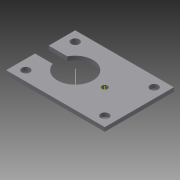
# Autodesk Inventor part: GehäuseFront
Saved by Autodesk Inventor 2014 (Build 180170000, 170)
## iProperties
Created: 2013-05-31
Part Number: GehäuseFront
Material: Generisch
Document SubType Name: Modeling
Designer: hanse
Density: 1 g/cm^3
Appearance: Vorgabe
Author: hanse
Autodesk Inventor part; units mm, degrees
ref_plane "YZ Plane" through (0, 0, 0) normal (1, 0, 0) x (0, 1, 0)
ref_plane "XZ Plane" through (0, 0, 0) normal (0, 1, 0) x (-1, 0, 0)
ref_plane "XY Plane" through (0, 0, 0) normal (0, 0, 1) x (1, 0, 0)
sketch "Skizze1" plane through (0, 0, 0) normal (0, 0, 1) x (1, 0, 0)
  line L0 (0, 0) -> (50, 0)
  line L1 (50, 0) -> (50, 35)
  line L2 (50, 35) -> (0, 35)
  line L3 (0, 35) -> (0, 0)
  circle A0 centre (17.5, 17.5) radius 1.05
  circle A1 centre (32.5, 17.5) radius 1.45
  line L4 (0, 17.5) -> (50, 17.5)
  line L5 (50, 0) -> (50, 17.5)
  line L6 (50, 17.5) -> (50, 35)
  line L7 (17.5, 17.5) -> (0, 17.5)
  line L8 (32.5, 17.5) -> (50, 17.5)
  dimension "d0" = 2.1
  dimension "d1" = 2.9
  dimension "d2" = 15
  dimension "d16" = 17.5
  dimension "d25" = 50
  constraints: 18 end point, 6 collinear, 2 centre point, 2 midpoint, 2 parallel, 2 perpendicular, 2 point on line, 1 horizontal
  measures "d0" diameter of A0
  measures "d1" diameter of A1
  measures "d2" distance of L8.start L7.start
  measures "d16" distance between parallel lines of L2 L4
  measures "d25" distance of L0.start L0.end
extrude "Extrusion1" add sketch "Skizze1" along normal blind 2 contours L3 L4 A0 A1 L1 L0 | L3 L2 L1 L4 A1 A0
sketch "Skizze5" plane through (0, 0, 2) normal (0, 0, 1) x (1, 0, 0)
  circle A0 centre (17.5, 17.5) radius 1.05 projected
  circle A1 centre (17.5, 17.5) radius 9
  line L0 (10.0196, 14.6319) -> (-2.5086, 14.6319)
  line L1 (-2.5086, 14.6319) -> (-2.5086, 21.5511)
  line L2 (-2.5086, 21.5511) -> (10.0196, 21.5511)
  line L3 (10.0196, 21.5511) -> (10.0196, 14.6319)
  circle A2 centre (17.5, 17.5) radius 7.5 projected
  dimension "d24" = 1.5
  constraints: 8 end point, 2 parallel, 1 centre point, 1 coincident, 1 horizontal, 1 perpendicular
  measures "d24" radial gap between concentric circles of A1 A2
extrude "Extrusion5" cut sketch "Skizze5" against normal through all
sketch "Skizze6" plane through (0, 0, 2) normal (0, 0, 1) x (1, 0, 0)
  line L0 (0, 14.6319) -> (0, 0) projected
  line L1 (0, 0) -> (50, 0) projected
  line L2 (50, 0) -> (50, 35) projected
  line L3 (50, 35) -> (0, 35) projected
  line L4 (5, 30) -> (45, 30)
  line L5 (45, 30) -> (45, 5)
  line L6 (45, 5) -> (5, 5)
  line L7 (5, 5) -> (5, 30)
  dimension "d26" = 5
  dimension "d27" = 5
  dimension "d28" = 5
  dimension "d29" = 5
  constraints: 8 end point, 2 parallel, 1 horizontal, 1 perpendicular
  measures "d26" distance between parallel lines of L3 L4
  measures "d27" distance between parallel lines of L6 L1
  measures "d28" distance between parallel lines of L0 L7
  measures "d29" distance between parallel lines of L2 L5
hole "Bohrung1" at (5, 5, 2) at (5, 30, 2) at (45, 30, 2) at (45, 5, 2) direction (0, 0, -1) diameter 4.1 end through all
